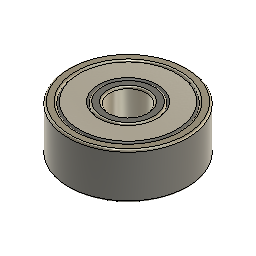
3_Assembly - Connection_Suspension v35 (Autodesk Fusion 360 archive; units mm, degrees)
design "Rolling 4x13x5"
Autodesk Fusion 360 part; units mm, degrees
sketch "Sketch1" plane through (0, 0, 0) normal (0, 0, 1) x (1, 0, 0)
  circle A0 centre (0, 0) radius 6.5
  circle A1 centre (0, 0) radius 2
  circle A2 centre (0, 0) radius 5.5
  circle A3 centre (0, 0) radius 3
  dimension "d1" = 13
  dimension "d2" = 4
  dimension "d5" = -1
  dimension "d6" = 1
  constraint coincident A0.centre A1.centre
  measures "d1" diameter of A0
  measures "d2" diameter of A1
extrude "Extrude2" add sketch "Sketch1" along normal blind 5 contours A0 makes body 1
fillet "Fillet1" radius 0.2 2 edges at (-6.0601, -2.3505, 5) (-5.1278, 1.9889, 5) on bodies 1
fillet "Fillet1" radius 0.2 2 edges at (-6.0601, -2.3505, 0) (-5.1278, 1.9889, 0) on bodies 1
extrude "Extrude3" add sketch "Sketch1" along normal blind 5 separate body contours A3 makes body 2
fillet "Fillet2" radius 0.2 2 edges at (-2.797, -1.0848, 5) (-1.8647, 0.7232, 5) on bodies 2
fillet "Fillet2" radius 0.2 2 edges at (-2.797, -1.0848, 0) (-1.8647, 0.7232, 0) on bodies 2
extrude "Extrude4" add sketch "Sketch1" along normal blind 5 separate body contours A2 makes body 3
fillet "Fillet3" radius 0.2 2 edges at (-5.1278, -1.9889, 5) (-2.797, 1.0848, 5) on bodies 3
fillet "Fillet3" radius 0.2 2 edges at (-5.1278, -1.9889, 0) (-2.797, 1.0848, 0) on bodies 3
combine "Combine1" operation add target body 1 tool bodies 2 3

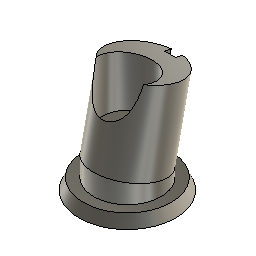
design "Bielle 2"
Autodesk Fusion 360 part; units mm, degrees
sketch "Sketch1" plane through (0, 0, 0) normal (0, 0, 1) x (1, 0, 0)
  circle A0 centre (0, 0) radius 16.75
  dimension "d1" = 33.5
  constraint coincident A0.centre origin
  measures "d1" diameter of A0
extrude "Extrude1" add sketch "Sketch1" along normal blind 11 makes body 1
sketch "Sketch2" plane through (0, 0, 11) normal (0, 0, 1) x (-1, 0, 0)
  circle A0 centre (0, 0) radius 16.75
  circle A1 centre (0, 0) radius 21.5
  dimension "d4" = 43
  constraint coincident A0.centre A1.centre
  measures "d4" diameter of A1
extrude "Extrude2" add sketch "Sketch2" along normal blind 5 contours A0 | A1 bodies 1
chamfer "Chamfer1" distance 2 distance2 5 1 edges at (20.045, 7.7747, 16) measured on face at (0.08, -1.0681, 16) on bodies 1
sketch "Sketch3" plane through (0, 0, 16) normal (0, 0, 1) x (-1, 0, 0)
  circle A0 centre (0, 0) radius 19.5
  circle A1 centre (0, 0) radius 15
  dimension "d10" = 30
  constraint coincident A0.centre A1.centre
  measures "d10" diameter of A1
extrude "Extrude3" add sketch "Sketch3" along normal blind 17 contours A1 bodies 1
ref_plane "WorkPlane1" through (12.125, 0, 0) normal (0, 0.207912, 0.978148) x (1, 0, 0)
ref_plane "WorkPlane2" through (12.125, 4.5117, 21.2258) normal (0, 0.207912, 0.978148) x (1, 0, 0)
split "Split1" by plane through (12.125, 4.5117, 21.2258) normal (0, 0.207912, 0.978148) bodies 1 makes body 2 at (-2.338, 14.8167, 28.3475)
extrude "Extrude4" add 1 faces at (4.9784, 0.274, 22.1265) along direction (0, 0.207912, 0.978148) blind 35 on bodies 1 bodies 1
sketch "Sketch7" plane through (0, 0, 0) normal (0, 0, -1) x (1, 0, 0)
  circle A0 centre (0, 0) radius 16.75
  circle A1 centre (0, 0) radius 5.25
  dimension "d33" = 10.5
  constraint coincident A0.centre A1.centre
  measures "d33" diameter of A1
extrude "Extrude9" cut sketch "Sketch7" against normal through all contours A1 bodies 1
ref_plane "WorkPlane3" through (0, 0, 62) normal (0, 0, 1) x (1, 0, 0)
sketch "Sketch8" plane through (0, 0, 62) normal (0, 0, 1) x (1, 0, 0)
  circle A0 centre (0, 0) radius 11.1
  dimension "d36" = 22.2
  constraint coincident A0.centre origin
  measures "d36" diameter of A0
extrude "Extrude10" cut sketch "Sketch8" against normal blind 28 bodies 1
ref_plane "WorkPlane4" through (0, 0, 11) normal (0, 0, -1) x (1, 0, 0)
split "Split2" by plane through (0, 0, 11) normal (0, 0, -1) bodies 1 makes body 3 at (16.7292, -0.8349, 7.3333)
sketch "Sketch9" plane through (0, 0, 11) normal (0, 0, -1) x (1, 0, 0)
  circle A0 centre (0, 0) radius 4.5
  circle A1 centre (0, 0) radius 16.75
  line L0 (10.1, 5.8312) -> (0, 11.6625)
  line L1 (0, 11.6625) -> (-10.1, 5.8312)
  line L2 (-10.1, 5.8312) -> (-10.1, -5.8312)
  line L3 (-10.1, -5.8312) -> (0, -11.6625)
  line L4 (0, -11.6625) -> (10.1, -5.8312)
  line L5 (10.1, -5.8312) -> (10.1, 5.8312)
  circle A2 centre (0, 0) radius 21.5
  circle A3 centre (0, 0) radius 5.25
  dimension "d51" = 10.1
  constraint coincident A0.centre A1.centre
  measures "d51" distance of A0.centre L5
ref_plane "WorkPlane6" through (0, 2.99, 36.2518) normal (0, -0.978148, 0.207912) x (0, 0.207912, 0.978148)
ref_plane "WorkPlane7" through (0, 12.7715, 34.1727) normal (0, -0.978148, 0.207912) x (0, 0.207912, 0.978148)
sketch "Sketch10" plane through (0, 12.7715, 34.1727) normal (0, -0.978148, 0.207912) x (0, 0.207912, 0.978148)
  line L0 (20.6187, -15) -> (20.6187, 15)
  line L1 (-14.3813, -15) -> (-14.3813, 15)
  line L2 (-14.3813, -15) -> (-14.3813, 15)
  line L3 (20.6187, 15) -> (-14.3813, -15) construction
  line L4 (20.6187, 0) -> (-14.3813, 0) construction
  line L5 (20.6187, -2.5) -> (-14.3813, -2.5)
  line L6 (-14.3813, -2.5) -> (-14.3813, 2.5)
  line L7 (-14.3813, 2.5) -> (20.6187, 2.5)
  line L8 (20.6187, 2.5) -> (20.6187, -2.5)
  dimension "d58" = 5
  constraint coincident L0.end L3.start
  constraint coincident L1.start L2.start
  constraint midpoint L0 L4.start
  constraint midpoint L2 L4.end
  constraint horizontal L5
  constraint vertical L6
  constraint horizontal L7
  constraint vertical L8
  constraint coincident L1 L6.end
  constraint coincident L0 L5.start
  constraint midpoint L4.start L8
  measures "d58" distance of L5.start L7.end
extrude "Extrude14" add sketch "Sketch10" against normal blind 7 bodies 1
extrude "Extrude11" cut sketch "Sketch9" against normal blind 11 contours L0 L1 L2 L3 L4 L5 bodies 1
extrude "Extrude17" cut 1 faces at (0.8333, 21.4798, 41.4737) along direction (0, -0.978148, 0.207912) blind 5 on bodies 1 bodies 1
extrude "Extrude18" add 1 faces at (0.2789, 12.8174, 19.4604) along direction (0, 0.207912, 0.978148) blind 3 on bodies 1 bodies 1
sketch "Sketch12" plane through (0, 0, 34) normal (0, 0, 1) x (-1, 0, 0)
  circle A0 centre (0, 0) radius 5.25
  circle A1 centre (0, 0) radius 11.1
  circle A2 centre (0, 0) radius 6.5
  dimension "d73" = 13
  constraint coincident A0.centre A1.centre
  measures "d73" diameter of A2
extrude "Extrude19" [rolled back] along distance -1 taper angle 0
hidden bodies 2 3

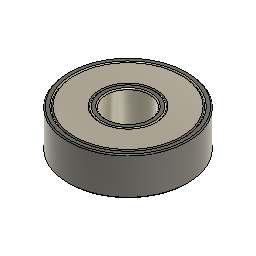
design "Rolling"
Autodesk Fusion 360 part; units mm, degrees
sketch "Sketch1" plane through (0, 0, 0) normal (0, 0, 1) x (1, 0, 0)
  circle A0 centre (0, 0) radius 11
  circle A1 centre (0, 0) radius 4
  circle A2 centre (0, 0) radius 10
  circle A3 centre (0, 0) radius 5
  dimension "d1" = 22
  dimension "d2" = 8
  dimension "d5" = -1
  dimension "d6" = 1
  constraint coincident A0.centre A1.centre
  measures "d1" diameter of A0
  measures "d2" diameter of A1
extrude "Extrude2" add sketch "Sketch1" along normal blind 7 contours A0 makes body 1
fillet "Fillet1" radius 0.2 2 edges at (-10.2556, -3.9778, 7) (-9.3233, 3.6162, 7) on bodies 1
fillet "Fillet1" radius 0.2 2 edges at (-10.2556, -3.9778, 0) (-9.3233, 3.6162, 0) on bodies 1
extrude "Extrude3" add sketch "Sketch1" along normal blind 7 separate body contours A3 makes body 2
fillet "Fillet2" radius 0.2 2 edges at (-4.6616, -1.8081, 7) (-3.7293, 1.4465, 7) on bodies 2
fillet "Fillet2" radius 0.2 2 edges at (-4.6616, -1.8081, 0) (-3.7293, 1.4465, 0) on bodies 2
extrude "Extrude4" add sketch "Sketch1" along normal blind 7 separate body contours A2 makes body 3
fillet "Fillet3" radius 0.2 2 edges at (-9.3233, -3.6162, 7) (-4.6616, 1.8081, 7) on bodies 3
fillet "Fillet3" radius 0.2 2 edges at (-9.3233, -3.6162, 0) (-4.6616, 1.8081, 0) on bodies 3
combine "Combine1" operation add target body 1 tool bodies 2 3

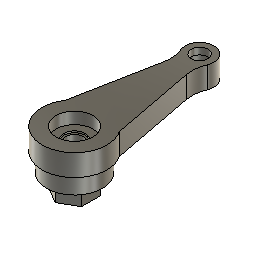
design "Bielle"
Autodesk Fusion 360 part; units mm, degrees
sketch "Sketch1" plane through (0, 0, 0) normal (0, 0, 1) x (1, 0, 0)
  circle A0 centre (0, 0) radius 18 construction
  line L0 (-3.7812, 75.9244) -> (-17.6785, 3.387)
  circle A1 centre (0, 75.2) radius 3.85 construction
  circle A2 centre (0, 0) radius 19.5
  line L1 (17.6785, 3.387) -> (3.7812, 75.9244)
  line L2 (0, 0) -> (0, 100) construction
  circle A3 centre (0, 75.2) radius 8.6
  circle A4 centre (0, 0) radius 11.1
  circle A5 centre (0, 0) radius 5.25
  dimension "d2" = 39
  dimension "d3" = 36
  dimension "d4" = 7.7
  dimension "d5" = 75.2
  dimension "d15" = 22.2
  dimension "d16" = 10.5
  constraint coincident L0.end A0
  constraint coincident L0.start A1
  constraint coincident A0.centre A2.centre
  constraint coincident A0 L1.start
  constraint coincident A1 L1.end
  constraint tangent A1 L1
  constraint tangent A0 L1
  constraint tangent A0 L0
  constraint tangent L0 A1
  constraint vertical L2
  constraint coincident A1.centre L2
  measures "d2" diameter of A2
  measures "d3" diameter of A0
  measures "d4" diameter of A1
  measures "d5" distance of A0.centre A1.centre
  measures "d15" diameter of A4
  measures "d16" diameter of A5
extrude "Extrude1" add sketch "Sketch1" along normal blind 13 contours L0 A2 L1 A3 | A3 | A2
extrude "Extrude4" add sketch "Sketch1" along normal blind 6 contours A4
extrude "Extrude5" add sketch "Sketch1" along normal blind 4 contours L0 A2 L1 A3
fillet "Fillet2" radius 20 2 edges at (-5.2282, 68.3717, 6.5) (5.2282, 68.3717, 6.5)
sketch "Sketch2" plane through (0, 0, 0) normal (0, 0, -1) x (1, 0, 0)
  arc A0 (6.7512, -60.4223) -> (7.9367, -71.888) centre (26.394, -64.1856) ccw
  line L0 (6.7512, -60.4223) -> (16.2672, -10.753)
  arc A1 (16.2672, -10.753) -> (-16.2672, -10.753) centre (0, 0) ccw
  line L1 (-16.2672, -10.753) -> (-6.7512, -60.4223)
  arc A2 (-7.9367, -71.888) -> (-6.7512, -60.4223) centre (-26.394, -64.1856) ccw
  arc A3 (-7.9367, -71.888) -> (7.9367, -71.888) centre (0, -75.2) ccw
  circle A4 centre (0, 0) radius 16.75
  circle A5 centre (0, 0) radius 5.25
  circle A6 centre (0, 0) radius 4.5
  dimension "d27" = 33.5
  constraint coincident A1.centre A4.centre
  constraint concentric A4 A6
  measures "d27" diameter of A4
extrude "Extrude6" add sketch "Sketch2" along normal blind 11 contours A4
sketch "Sketch3" plane through (0, 0, -11) normal (0, 0, -1) x (1, 0, 0)
  circle A0 centre (0, 0) radius 5.25
  circle A1 centre (0, 0) radius 16.75
  line L0 (10, 5.7735) -> (0, 11.547)
  line L1 (0, 11.547) -> (-10, 5.7735)
  line L2 (-10, 5.7735) -> (-10, -5.7735)
  line L3 (-10, -5.7735) -> (0, -11.547)
  line L4 (0, -11.547) -> (10, -5.7735)
  line L5 (10, -5.7735) -> (10, 5.7735)
  constraint coincident A0.centre A1.centre
extrude "Extrude7" add sketch "Sketch3" along normal blind 10 contours L0 L1 L2 L3 L4 L5
sketch "Sketch4" plane through (0, 0, 0) normal (0, 0, -1) x (1, 0, 0)
  circle A0 centre (0, 0) radius 16.75
  arc A1 (6.7512, -60.4223) -> (7.9367, -71.888) centre (26.394, -64.1856) ccw
  line L0 (6.7512, -60.4223) -> (16.2672, -10.753)
  arc A2 (16.2672, -10.753) -> (-16.2672, -10.753) centre (0, 0) ccw
  line L1 (-16.2672, -10.753) -> (-6.7512, -60.4223)
  arc A3 (-7.9367, -71.888) -> (-6.7512, -60.4223) centre (-26.394, -64.1856) ccw
  arc A4 (-7.9367, -71.888) -> (7.9367, -71.888) centre (0, -75.2) ccw
  circle A5 centre (0, -75.2) radius 6.55
  circle A6 centre (0, -75.2) radius 5
  dimension "d32" = 13.1
  dimension "d33" = 10
  constraint concentric A4 A5
  constraint concentric A5 A6
  measures "d32" diameter of A5
  measures "d33" diameter of A6
extrude "Extrude8" cut sketch "Sketch4" against normal through all contours A6
extrude "Extrude9" cut sketch "Sketch4" against normal blind 9 contours A5
sketch "Sketch5" plane through (0, 0, 6) normal (0, 0, 1) x (-1, 0, 0)
  circle A0 centre (0, 0) radius 5.25
  circle A1 centre (0, 0) radius 11.1
  circle A2 centre (0, 0) radius 6.5
  dimension "d37" = 13
  constraint concentric A0 A2
  measures "d37" diameter of A2
extrude "Extrude10" cut sketch "Sketch5" against normal blind 1 contours A2
equation "d20 = 13 mm - 7 mm"
equation "d22 = ( ( 13 / 2 ) * 1 mm ) - 2.5 mm"
